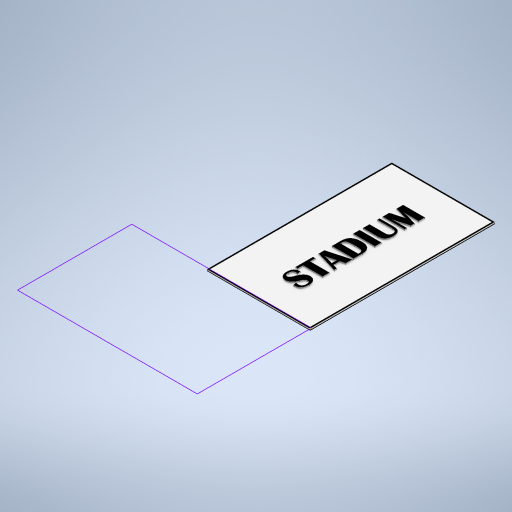
# Autodesk Inventor part: banner2
Saved by Autodesk Inventor 2024.1 (Build 281209000, 209)
## iProperties
Created: 2023-11-18
Part Number: banner2
Material: Generic
Document SubType Name: Modeling
Designer: ASUS
Density: 1 g/cm^3
Appearance: Default
Author: ASUS
Autodesk Inventor part; units mm, degrees
ref_plane "YZ Plane" through (0, 0, 0) normal (1, 0, 0) x (0, 1, 0)
ref_plane "XZ Plane" through (0, 0, 0) normal (0, 1, 0) x (-1, 0, 0)
ref_plane "XY Plane" through (0, 0, 0) normal (0, 0, 1) x (1, 0, 0)
sketch "Sketch1" plane through (0, 0, 0) normal (0, 1, 0) x (-1, 0, 0)
  line L0 (0, 0) -> (19812, 0)
  line L1 (19812, 0) -> (19812, -35560)
  line L2 (19812, -35560) -> (0, -35560)
  line L3 (0, -35560) -> (0, 0)
  line L4 (19558, -35306) -> (19558, -254)
  line L5 (19558, -254) -> (254, -254)
  line L6 (254, -254) -> (254, -35306)
  line L7 (254, -35306) -> (19558, -35306)
  line L8 (11476.6644, -5257.4578) -> (11476.6644, -18725.3039) construction
  line L9 (11476.6644, -18725.3039) -> (-12932.071, -18725.3039) construction
  line L10 (-12932.071, -18725.3039) -> (-12932.071, -5257.4578) construction
  line L11 (-12932.071, -5257.4578) -> (11476.6644, -5257.4578) construction
  line L12 (10240.4018, -8337.9814) -> (10139.0688, -7777.272)
  spline S0 degree 2 poles (10139.0688, -7777.272) (10304.5794, -7814.4275) (10419.4235, -7814.4275) knots 0 0 0 1 1 1
  spline S1 degree 2 poles (10419.4235, -7814.4275) (11145.6434, -7814.4275) (11145.6434, -6932.8303) knots 0 0 0 1 1 1
  spline S2 degree 2 poles (11145.6434, -6932.8303) (11145.6434, -6237.0103) (10645.7338, -6237.0103) knots 0 0 0 1 1 1
  spline S3 degree 2 poles (10645.7338, -6237.0103) (10270.8017, -6237.0103) (10000.5803, -7013.8967) knots 0 0 0 1 1 1
  spline S4 degree 2 poles (10000.5803, -7013.8967) (9487.1597, -8513.6252) (8477.2074, -8513.6252) knots 0 0 0 1 1 1
  spline S5 degree 2 poles (8477.2074, -8513.6252) (7882.7204, -8513.6252) (7166.6338, -7672.5613) (7166.6338, -6973.3635) knots 0 0 0 1 2 2 2
  spline S6 degree 2 poles (7166.6338, -6973.3635) (7166.6338, -5429.7239) (8365.7411, -5429.7239) knots 0 0 0 1 1 1
  spline S7 degree 2 poles (8365.7411, -5429.7239) (8463.6963, -5429.7239) (8608.9403, -5443.235) knots 0 0 0 1 1 1
  line L13 (8608.9403, -5443.235) -> (8733.9177, -6027.5887)
  spline S8 degree 2 poles (8733.9177, -6027.5887) (8470.4519, -5960.0334) (8274.5414, -5960.0334) knots 0 0 0 1 1 1
  spline S9 degree 2 poles (8274.5414, -5960.0334) (7497.655, -5960.0334) (7497.655, -6848.3861) knots 0 0 0 1 1 1
  spline S10 degree 2 poles (7497.655, -6848.3861) (7497.655, -7557.7172) (8054.9865, -7557.7172) knots 0 0 0 1 1 1
  spline S11 degree 2 poles (8054.9865, -7557.7172) (8470.4519, -7557.7172) (8784.5842, -6706.5199) knots 0 0 0 1 1 1
  spline S12 degree 2 poles (8784.5842, -6706.5199) (9237.205, -5477.0127) (10230.2685, -5477.0127) knots 0 0 0 1 1 1
  spline S13 degree 2 poles (10230.2685, -5477.0127) (10790.9778, -5477.0127) (11476.6645, -6297.8101) (11476.6645, -6966.6079) knots 0 0 0 1 2 2 2
  spline S14 degree 2 poles (11476.6645, -6966.6079) (11476.6645, -8337.9814) (10240.4018, -8337.9814) knots 0 0 0 1 1 1
  line L14 (11405.7314, -11965.7032) -> (10986.8883, -11965.7032)
  line L15 (10986.8883, -11965.7032) -> (10986.8883, -10945.6175)
  line L16 (10986.8883, -10945.6175) -> (7244.3224, -10945.6175)
  line L17 (7244.3224, -10945.6175) -> (7244.3224, -9665.4438)
  line L18 (7244.3224, -9665.4438) -> (10986.8883, -9665.4438)
  line L19 (10986.8883, -9665.4438) -> (10986.8883, -8638.6026)
  line L20 (10986.8883, -8638.6026) -> (11405.7314, -8638.6026)
  line L21 (11405.7314, -8638.6026) -> (11405.7314, -11965.7032)
  line L22 (11405.7314, -14171.385) -> (7244.3224, -15329.9591)
  line L23 (7244.3224, -15329.9591) -> (7244.3224, -14117.3408)
  line L24 (7244.3224, -14117.3408) -> (8146.1862, -13870.7638)
  line L25 (8146.1862, -13870.7638) -> (8146.1862, -12617.6122)
  line L26 (8146.1862, -12617.6122) -> (7244.3224, -12350.7686)
  line L27 (7244.3224, -12350.7686) -> (7244.3224, -11877.8812)
  line L28 (7244.3224, -11877.8812) -> (11405.7314, -13110.7662)
  line L29 (11405.7314, -13110.7662) -> (11405.7314, -14171.385)
  line L30 (8565.0293, -12735.8341) -> (8565.0293, -13759.2975)
  line L31 (8565.0293, -13759.2975) -> (10409.2902, -13266.1435)
  line L32 (10409.2902, -13266.1435) -> (8565.0293, -12735.8341)
  line L33 (7244.3224, -15657.6025) -> (11405.7314, -15657.6025)
  line L34 (11405.7314, -15657.6025) -> (11405.7314, -17383.6415)
  spline S15 degree 2 poles (11405.7314, -17383.6415) (11405.7314, -19224.5245) (9321.6492, -19224.5245) knots 0 0 0 1 1 1
  spline S16 degree 2 poles (9321.6492, -19224.5245) (7244.3224, -19224.5245) (7244.3224, -17319.4639) knots 0 0 0 1 1 1
  line L35 (7244.3224, -17319.4639) -> (7244.3224, -15657.6025)
  line L36 (7588.8547, -16866.8431) -> (7588.8547, -17184.3532)
  spline S17 degree 2 poles (7588.8547, -17184.3532) (7588.8547, -17620.0852) (8342.0967, -17954.4841) (9325.0269, -17954.4841) knots 0 0 0 1 2 2 2
  spline S18 degree 2 poles (9325.0269, -17954.4841) (10311.3349, -17954.4841) (11061.1992, -17623.463) (11061.1992, -17184.3532) knots 0 0 0 1 2 2 2
  line L37 (11061.1992, -17184.3532) -> (11061.1992, -16866.8431)
  line L38 (11061.1992, -16866.8431) -> (7588.8547, -16866.8431)
  line L39 (11405.7314, -20964.0746) -> (7244.3224, -20964.0746)
  line L40 (7244.3224, -20964.0746) -> (7244.3224, -19754.834)
  line L41 (7244.3224, -19754.834) -> (11405.7314, -19754.834)
  line L42 (11405.7314, -19754.834) -> (11405.7314, -20964.0746)
  line L43 (11405.7314, -24814.729) -> (8612.3181, -24814.729)
  spline S19 degree 2 poles (8612.3181, -24814.729) (7176.7671, -24814.729) (7176.7671, -23227.1785) knots 0 0 0 1 1 1
  spline S20 degree 2 poles (7176.7671, -23227.1785) (7176.7671, -21643.0057) (8612.3181, -21643.0057) knots 0 0 0 1 1 1
  line L44 (8612.3181, -21643.0057) -> (11405.7314, -21643.0057)
  line L45 (11405.7314, -21643.0057) -> (11405.7314, -22852.2463)
  line L46 (11405.7314, -22852.2463) -> (8578.5404, -22852.2463)
  spline S21 degree 2 poles (8578.5404, -22852.2463) (8027.9644, -22852.2463) (7626.0101, -23166.3787) (7626.0101, -23588.5996) knots 0 0 0 1 2 2 2
  spline S22 degree 2 poles (7626.0101, -23588.5996) (7626.0101, -24409.397) (8612.3181, -24409.397) knots 0 0 0 1 1 1
  line L47 (8612.3181, -24409.397) -> (11405.7314, -24409.397)
  line L48 (11405.7314, -24409.397) -> (11405.7314, -24814.729)
  line L49 (11405.7314, -29334.1813) -> (7244.3224, -29334.1813)
  line L50 (7244.3224, -29334.1813) -> (7244.3224, -28168.8517)
  line L51 (7244.3224, -28168.8517) -> (10142.4466, -28168.8517)
  line L52 (10142.4466, -28168.8517) -> (7244.3224, -27358.1876)
  line L53 (7244.3224, -27358.1876) -> (7244.3224, -26682.6342)
  line L54 (7244.3224, -26682.6342) -> (10091.78, -25851.7035)
  line L55 (10091.78, -25851.7035) -> (7244.3224, -25851.7035)
  line L56 (7244.3224, -25851.7035) -> (7244.3224, -25446.3714)
  line L57 (7244.3224, -25446.3714) -> (11405.7314, -25446.3714)
  line L58 (11405.7314, -25446.3714) -> (11405.7314, -26672.5009)
  line L59 (11405.7314, -26672.5009) -> (8892.6727, -27385.2097)
  line L60 (8892.6727, -27385.2097) -> (11405.7314, -28094.5408)
  line L61 (11405.7314, -28094.5408) -> (11405.7314, -29334.1813)
  constraints: 16 end point, 4 parallel, 2 perpendicular, 1 horizontal, 5 other
extrude "Extrusion1" add sketch "Sketch1" along normal blind 508 contours L12 S0 S1 S2 S3 S4 S5 S6 S7 L13 S8 S9 S10 S11 S12 S13 S14 | L14 L15 L16 L17 L18 L19 L20 L21 | L22 L23 L24 L25 L26 L27 L28 L29 | L33 L34 S15 S16 L35 | L39 L40 L41 L42 | L43 S19 S20 L44 L45 L46 S21 S22 L47 L48 | L49 L50 L51 L52 L53 L54 L55 L56 L57 L58 L59 L60 L61
extrude "Extrusion2" add sketch "Sketch1" along normal blind 254 separate body contours L7 L6 L5 L4 | L12 S0 S1 S2 S3 S4 S5 S6 S7 L13 S8 S9 S10 S11 S12 S13 S14 | L14 L15 L16 L17 L18 L19 L20 L21 | L22 L23 L24 L25 L26 L27 L28 L29 | L32 L31 L30 | L33 L34 S15 S16 L35 | L38 L37 S18 S17 L36 | L39 L40 L41 L42 | L43 S19 S20 L44 L45 L46 S21 S22 L47 L48 | L49 L50 L51 L52 L53 L54 L55 L56 L57 L58 L59 L60 L61
extrude "Extrusion3" add sketch "Sketch1" along normal blind 254 separate body contours L0 L1 L2 L3
sketch "Sketch2" plane through (0, 254, 0) normal (0, 1, 0) x (1, 0, 0)
  line L0 (0, 254) -> (-34633.9567, 254)
  line L1 (-34633.9567, 254) -> (-34633.9567, -21754.7824)
  line L2 (-34633.9567, -21754.7824) -> (0, -21754.7824)
  line L3 (0, -21754.7824) -> (0, 254)
  point P0 (0, 0)
  constraints: 8 end point, 2 parallel, 1 horizontal, 1 perpendicular
body "Solid1"
body "Solid2"
body "Solid3"
